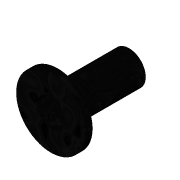
# Autodesk Inventor part: 50_ETL_Motionpart1_v0
Saved by Autodesk Inventor 2022 (Build 260153000, 153)
## iProperties
Created: 2021-12-31
Part Number: 50_ETL_Motionpart1_v0
Material: Generisch
Document SubType Name: Modeling
Designer: diederichbenedict
Density: 1 g/cm^3
Appearance: Schwarz
Author: diederichbenedict
Autodesk Inventor part; units mm, degrees
ref_plane "YZ Plane" through (0, 0, 0) normal (1, 0, 0) x (0, 1, 0)
ref_plane "Arbeitsebene2" through (-24.4207, -24.3793, -13.5) normal (0, 0, -1) x (0, 1, 0)
ref_plane "Arbeitsebene3" through (-24.4207, -24.3793, -18.5) normal (0, 0, -1) x (0, 1, 0)
sketch "Skizze1" plane through (0, 0, 0) normal (0, 0, 1) x (1, 0, 0)
  arc A0 (-2.8009, 5.3061) -> (2.8009, 5.3061) centre (0, 0) ccw projected
  circle A1 centre (0, 0) radius 5 projected
  circle A2 centre (0, 0) radius 4.8
  circle A3 centre (0, 0) radius 4.05
  circle A4 centre (0, 0) radius 10
  point P0 (0, 0)
  dimension "d0" = 0.2
  dimension "d1" = 8.1
  dimension "d14" = 20
  constraints: 3 centre point, 2 coincident
  measures "d0" radial gap between concentric circles of A1 A2
  measures "d1" diameter of A3
  measures "d14" diameter of A4
extrude "Extrusion1" add sketch "Skizze1" against normal up to surface (18.5 mm away) contours A2
sketch "Skizze2" plane through (0, 0, 0) normal (0, 0, 1) x (1, 0, 0)
  circle A0 centre (0, 0) radius 4.8 projected
  circle A1 centre (0, 0) radius 4.05 projected
  arc A2 (2.3233, 6.0706) -> (-5.9453, 2.6275) centre (0, 0) ccw projected
  circle A3 centre (0, 0) radius 6.5
  point P0 (-5.9453, 2.6275)
  point P1 (2.3233, 6.0706)
  constraints: 1 centre point, 1 coincident
extrude "Extrusion2" add sketch "Skizze2" along normal blind 2 contours A0 | A3 A2
sketch "Skizze4" plane through (0, 0, -18.5) normal (0, 0, -1) x (-1, 0, 0)
  circle A0 centre (0, 0) radius 4.05 projected
  circle A1 centre (0, 0) radius 1.4
  point P0 (0, 0)
  dimension "d16" = 2.8
  constraints: 1 centre point, 1 coincident
  measures "d16" diameter of A1
extrude "Extrusion4" add sketch "Skizze4" against normal blind 3
sketch "Skizze5" plane through (0, 0, 2) normal (0, 0, 1) x (1, 0, 0)
  circle A0 centre (0, 0) radius 6.5 projected
  circle A1 centre (0, 0) radius 6.5 projected
  circle A2 centre (0, 0) radius 4.05 projected
  circle A3 centre (0, 0) radius 10
  point P0 (0, 0)
  dimension "d19" = 20
  constraints: 1 centre point, 1 coincident
  measures "d19" diameter of A3
extrude "Extrusion5" add sketch "Skizze5" along normal blind 2 contours A0 | A3
